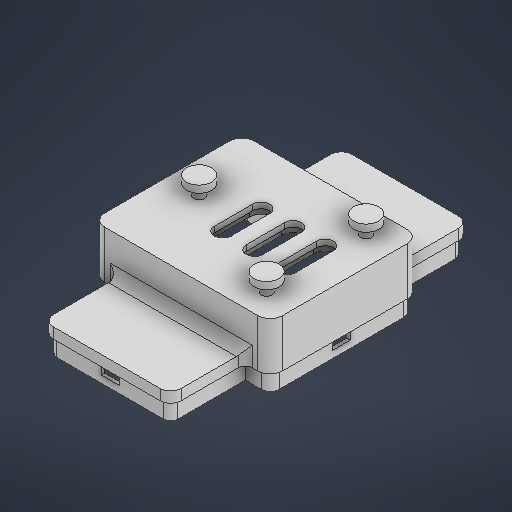
# Autodesk Inventor part: Body_Up
Saved by Autodesk Inventor 2026 (Build 300175000, 175)
## iProperties
Created: 2025-04-18
Part Number: Body_Up
Material: Generic
Document SubType Name: Modeling
Designer: ct_vi
Density: 1 g/cm^3
Appearance: Default
Author: ct_vi
Autodesk Inventor part; units mm, degrees
ref_plane "YZ Plane" through (0, 0, 0) normal (1, 0, 0) x (0, 1, 0)
ref_plane "XZ Plane" through (0, 0, 0) normal (0, 1, 0) x (-1, 0, 0)
ref_plane "XY Plane" through (0, 0, 0) normal (0, 0, 1) x (1, 0, 0)
sketch "Sketch1" plane through (0, 0, 0) normal (0, 1, 0) x (-1, 0, 0)
  line L0 (21.5, 21) -> (-21.5, 21)
  line L1 (-25, 17.5) -> (-25, -17.5)
  line L2 (-21.5, -21) -> (21.5, -21)
  line L3 (25, -17.5) -> (25, 17.5)
  line L4 (25, 21) -> (-25, -21) construction
  line L5 (-25, 21) -> (25, -21) construction
  line L6 (21.5, 20) -> (-21.5, 20)
  line L7 (-24, 17.5) -> (-24, -17.5)
  line L8 (-21.5, -20) -> (21.5, -20)
  line L9 (24, -17.5) -> (24, 17.5)
  line L10 (24, 20) -> (-24, -20) construction
  line L11 (-24, 20) -> (24, -20) construction
  line L12 (-21.5, 19) -> (21.5, 19)
  line L13 (23, 17.5) -> (23, -17.5)
  line L14 (21.5, -19) -> (-21.5, -19)
  line L15 (-23, -17.5) -> (-23, 17.5)
  line L16 (-23, 19) -> (23, -19) construction
  line L17 (23, 19) -> (-23, -19) construction
  line L18 (-22, 18) -> (22, -18) construction
  line L19 (22, 18) -> (-22, -18) construction
  line L20 (36.7273, 0) -> (-33.3361, 0)
  arc A0 (25, 17.5) -> (21.5, 21) centre (21.5, 17.5) ccw
  arc A1 (21.5, -21) -> (25, -17.5) centre (21.5, -17.5) ccw
  arc A2 (-21.5, 21) -> (-25, 17.5) centre (-21.5, 17.5) ccw
  arc A3 (-25, -17.5) -> (-21.5, -21) centre (-21.5, -17.5) ccw
  arc A4 (24, 17.5) -> (21.5, 20) centre (21.5, 17.5) ccw
  arc A5 (21.5, -20) -> (24, -17.5) centre (21.5, -17.5) ccw
  arc A6 (-21.5, 20) -> (-24, 17.5) centre (-21.5, 17.5) ccw
  arc A7 (-24, -17.5) -> (-21.5, -20) centre (-21.5, -17.5) ccw
  arc A8 (23, 17.5) -> (21.5, 19) centre (21.5, 17.5) ccw
  arc A9 (21.5, -19) -> (23, -17.5) centre (21.5, -17.5) ccw
  arc A10 (-23, -17.5) -> (-21.5, -19) centre (-21.5, -17.5) ccw
  arc A11 (-21.5, 19) -> (-23, 17.5) centre (-21.5, 17.5) ccw
  line L21 (-16, 20) -> (-16, 19)
  line L22 (16, 20) -> (16, 19)
  line L23 (-16, -20) -> (-16, -19)
  line L24 (16, -20) -> (16, -19)
  point P0 (0, 0)
  dimension "d0" = 50
  dimension "d1" = 42
  dimension "d2" = 48
  dimension "d3" = 40
  dimension "d4" = 46
  dimension "d5" = 38
  dimension "d27" = 3.5
  dimension "d28" = 2.5
  dimension "d29" = 1.5
  constraints: 50 end point, 29 point on line, 24 point on circle, 24 tangent, 12 centre point, 9 equal radius, 8 midpoint, 7 perpendicular, 6 parallel, 4 horizontal, 2 symmetric about line
  measures "d0" distance of L5.end L4.end
  measures "d1" distance of L4.end L5.start
  measures "d2" distance of L11.end L10.end
  measures "d3" distance of L10.end L11.start
  measures "d4" distance of L16.end L17.end
  measures "d5" distance of L17.start L16.end
  measures "d27" radius of A0
  measures "d28" radius of A4
  measures "d29" radius of A8
extrude "Extrusion1" add sketch "Sketch1" against normal blind 16 contours L20 L13 A8 L12 L22 L6 A4 L9 | L9 A5 L8 L24 L14 A9 L13 L20 | L20 L15 A10 L14 L23 L8 A7 L7 | L7 A6 L6 L21 L12 A11 L15 L20 | L8 L23 L14 L24 | L22 L12 L21 L6
extrude "Extrusion2" add sketch "Sketch1" along normal blind 2.5 and the other way blind 1
extrude "Extrusion5" add sketch "Sketch1" against normal blind 11 contours A0 L3 L20 L9 A4 L6 A6 L7 L1 A2 L0 | L3 A1 L2 A3 L1 L20 L7 A7 L8 A5 L9
sketch "Sketch7" plane through (0, -1, 0) normal (0, -1, 0) x (1, 0, 0)
  line L0 (14, -8.55) -> (14, -8.55)
  line L1 (17.15, -5.4) -> (17.15, 5.4)
  line L2 (14, 8.55) -> (14, 8.55)
  line L3 (10.85, 5.4) -> (10.85, -5.4)
  line L4 (10.85, -8.55) -> (17.15, 8.55) construction
  line L5 (17.15, -8.55) -> (10.85, 8.55) construction
  line L6 (5, -8.5739) -> (5, -8.5739)
  line L7 (8.15, -5.4239) -> (8.15, 5.3761)
  line L8 (5, 8.5261) -> (5, 8.5261)
  line L9 (1.85, 5.3761) -> (1.85, -5.4239)
  line L10 (1.85, -8.5739) -> (8.15, 8.5261) construction
  line L11 (8.15, -8.5739) -> (1.85, 8.5261) construction
  line L12 (5, -0.0239) -> (-4, -0.0239)
  line L13 (-4, -8.5739) -> (-4, -8.5739)
  line L14 (-0.85, -5.4239) -> (-0.85, 5.3761)
  line L15 (-4, 8.5261) -> (-4, 8.5261)
  line L16 (-7.15, 5.3761) -> (-7.15, -5.4239)
  line L17 (-7.15, -8.5739) -> (-0.85, 8.5261) construction
  line L18 (-0.85, -8.5739) -> (-7.15, 8.5261) construction
  arc A0 (-7.15, -5.4239) -> (-4, -8.5739) centre (-4, -5.4239) ccw
  arc A1 (-4, -8.5739) -> (-0.85, -5.4239) centre (-4, -5.4239) ccw
  arc A2 (-4, 8.5261) -> (-7.15, 5.3761) centre (-4, 5.3761) ccw
  arc A3 (-0.85, 5.3761) -> (-4, 8.5261) centre (-4, 5.3761) ccw
  arc A4 (1.85, -5.4239) -> (5, -8.5739) centre (5, -5.4239) ccw
  arc A5 (5, -8.5739) -> (8.15, -5.4239) centre (5, -5.4239) ccw
  arc A6 (8.15, 5.3761) -> (5, 8.5261) centre (5, 5.3761) ccw
  arc A7 (5, 8.5261) -> (1.85, 5.3761) centre (5, 5.3761) ccw
  arc A8 (10.85, -5.4) -> (14, -8.55) centre (14, -5.4) ccw
  arc A9 (14, -8.55) -> (17.15, -5.4) centre (14, -5.4) ccw
  arc A10 (17.15, 5.4) -> (14, 8.55) centre (14, 5.4) ccw
  arc A11 (14, 8.55) -> (10.85, 5.4) centre (14, 5.4) ccw
  line L19 (-4, 7.7261) -> (-4, 7.7261)
  line L20 (-1.65, 5.3761) -> (-1.65, -5.4239)
  line L21 (-4, -7.7739) -> (-4, -7.7739)
  line L22 (-6.35, -5.4239) -> (-6.35, 5.3761)
  line L23 (-6.35, 7.7261) -> (-1.65, -7.7739) construction
  line L24 (-1.65, 7.7261) -> (-6.35, -7.7739) construction
  line L25 (5, -7.7739) -> (5, -7.7739)
  line L26 (7.35, -5.4239) -> (7.35, 5.3761)
  line L27 (5, 7.7261) -> (5, 7.7261)
  line L28 (2.65, 5.3761) -> (2.65, -5.4239)
  line L29 (2.65, -7.7739) -> (7.35, 7.7261) construction
  line L30 (7.35, -7.7739) -> (2.65, 7.7261) construction
  line L31 (14, -7.75) -> (14, -7.75)
  line L32 (16.35, -5.4) -> (16.35, 5.4)
  line L33 (14, 7.75) -> (14, 7.75)
  line L34 (11.65, 5.4) -> (11.65, -5.4)
  line L35 (11.65, -7.75) -> (16.35, 7.75) construction
  line L36 (16.35, -7.75) -> (11.65, 7.75) construction
  arc A12 (-6.35, -5.4239) -> (-4, -7.7739) centre (-4, -5.4239) ccw
  arc A13 (-4, -7.7739) -> (-1.65, -5.4239) centre (-4, -5.4239) ccw
  arc A14 (-1.65, 5.3761) -> (-4, 7.7261) centre (-4, 5.3761) ccw
  arc A15 (-4, 7.7261) -> (-6.35, 5.3761) centre (-4, 5.3761) ccw
  arc A16 (2.65, -5.4239) -> (5, -7.7739) centre (5, -5.4239) ccw
  arc A17 (5, -7.7739) -> (7.35, -5.4239) centre (5, -5.4239) ccw
  arc A18 (7.35, 5.3761) -> (5, 7.7261) centre (5, 5.3761) ccw
  arc A19 (5, 7.7261) -> (2.65, 5.3761) centre (5, 5.3761) ccw
  arc A20 (11.65, -5.4) -> (14, -7.75) centre (14, -5.4) ccw
  arc A21 (14, -7.75) -> (16.35, -5.4) centre (14, -5.4) ccw
  arc A22 (16.35, 5.4) -> (14, 7.75) centre (14, 5.4) ccw
  arc A23 (14, 7.75) -> (11.65, 5.4) centre (14, 5.4) ccw
  point P0 (14, 0)
  point P1 (-4, -0.0239)
  point P2 (5, 8.5261)
  dimension "d99" = 6.3
  dimension "d100" = 17.1
  dimension "d102" = 6.3
  dimension "d103" = 17.1
  dimension "d105" = 9
  dimension "d106" = 6.3
  dimension "d107" = 17.1
  dimension "d108" = 3.15
  dimension "d109" = 4.7
  dimension "d110" = 15.5
  dimension "d111" = 4.7
  dimension "d112" = 15.5
  dimension "d113" = 4.7
  dimension "d114" = 15.5
  dimension "d115" = 2.35
  constraints: 74 end point, 48 point on circle, 48 point on line, 48 tangent, 24 centre point, 22 equal radius, 12 parallel, 10 midpoint, 7 horizontal, 6 perpendicular
  measures "d99" distance of L5.end L4.end
  measures "d100" distance of L4.end L5.start
  measures "d102" distance of L11.end L10.end
  measures "d103" distance of L10.end L11.start
  measures "d105" distance of L12.start L12.end
  measures "d106" distance of L18.end L17.end
  measures "d107" distance of L17.end L18.start
  measures "d108" radius of A0
  measures "d109" distance of L23.end L24.end
  measures "d110" distance of L24.start L23.end
  measures "d111" distance of L30.end L29.end
  measures "d112" distance of L29.end L30.start
  measures "d113" distance of L36.end L35.end
  measures "d114" distance of L35.end L36.start
  measures "d115" radius of A12
ref_plane "Work Plane4" through (0, -8, 0) normal (0, -1, 0) x (1, 0, 0)
sketch "Sketch11" plane through (0, -8, 0) normal (0, -1, 0) x (1, 0, 0)
  line L0 (0, 42) -> (-15, 42)
  line L1 (0, 42) -> (0, 41)
  line L2 (0, 41) -> (-15, 41)
  line L3 (0, 41) -> (0, 40)
  line L4 (0, 40) -> (-15, 40)
  line L5 (-18, 39) -> (-18, 20)
  line L6 (-17, 39) -> (-17, 20)
  line L7 (-16, 39) -> (-16, 19)
  line L8 (0, 21) -> (0, 42)
  line L9 (-18, 20) -> (0, 20)
  arc A0 (-15, 40) -> (-16, 39) centre (-15, 39) ccw
  arc A1 (-15, 41) -> (-17, 39) centre (-15, 39) ccw
  arc A2 (-15, 42) -> (-18, 39) centre (-15, 39) ccw
  line L10 (0, 0) -> (0, 21)
  line L11 (-16, 19) -> (0, 19)
  line L12 (-17, 20) -> (-17, 19)
  line L13 (-17, 19) -> (-16, 19)
  line L14 (-0.3234, 0) -> (-24.4289, 0)
  line L15 (-17, -19) -> (-16, -19)
  line L16 (-16, -19) -> (0, -19)
  line L17 (-17, -20) -> (-17, -19)
  line L18 (-18, -20) -> (0, -20)
  line L19 (-16, -39) -> (-16, -19)
  line L20 (-17, -39) -> (-17, -20)
  line L21 (-18, -39) -> (-18, -20)
  arc A3 (-17, -39) -> (-15, -41) centre (-15, -39) ccw
  arc A4 (-18, -39) -> (-15, -42) centre (-15, -39) ccw
  line L22 (0, -40) -> (-15, -40)
  line L23 (0, -41) -> (-15, -41)
  line L24 (0, -42) -> (0, -41)
  line L25 (0, -42) -> (-15, -42)
  arc A5 (-16, -39) -> (-15, -40) centre (-15, -39) ccw
  line L26 (17, -19) -> (16, -19)
  line L27 (17, -20) -> (17, -19)
  line L28 (16, -19) -> (0, -19)
  line L29 (18, -20) -> (0, -20)
  line L30 (16, -39) -> (16, -19)
  line L31 (18, -39) -> (18, -20)
  line L32 (17, -39) -> (17, -20)
  line L33 (0, 40) -> (15, 40)
  line L34 (0, 41) -> (15, 41)
  line L35 (0, 42) -> (15, 42)
  arc A6 (16, 39) -> (15, 40) centre (15, 39) ccw
  arc A7 (17, 39) -> (15, 41) centre (15, 39) ccw
  arc A8 (18, 39) -> (15, 42) centre (15, 39) ccw
  line L36 (16, 39) -> (16, 19)
  line L37 (17, 39) -> (17, 20)
  line L38 (18, 39) -> (18, 20)
  line L39 (16, 19) -> (0, 19)
  line L40 (18, 20) -> (0, 20)
  line L41 (17, 19) -> (16, 19)
  line L42 (17, 20) -> (17, 19)
  line L43 (0, -40) -> (15, -40)
  line L44 (0, -41) -> (15, -41)
  line L45 (0, -42) -> (15, -42)
  arc A9 (15, -40) -> (16, -39) centre (15, -39) ccw
  arc A10 (15, -41) -> (17, -39) centre (15, -39) ccw
  arc A11 (15, -42) -> (18, -39) centre (15, -39) ccw
  line L46 (0, -41) -> (0, -40)
  point P0 (0, 0)
  point P1 (0, 0)
  point P2 (-18, 42)
  point P3 (-17, 41)
  point P4 (-16, 40)
  point P5 (-16, -40)
  point P6 (-17, -41)
  point P7 (-18, -42)
  point P8 (0, -21)
  point P9 (16, -40)
  point P10 (18, -42)
  point P11 (17, -41)
  point P12 (16, 40)
  point P13 (17, 41)
  point P14 (18, 42)
  point P15 (16, 20)
  point P16 (-16, 20)
  point P17 (16, -20)
  point P18 (-16, -20)
  dimension "d127" = 21
  dimension "d128" = 21
  dimension "d129" = 18
  dimension "d130" = 90
  dimension "d131" = 22
  dimension "d132" = 1
  dimension "d133" = 17
  dimension "d134" = 90
  dimension "d135" = 1
  dimension "d136" = 16
  dimension "d137" = 21
  dimension "d138" = 3
  dimension "d139" = 2
  dimension "d140" = 1
  constraints: 94 end point, 54 symmetric about line, 32 point on line, 24 point on circle, 12 centre point, 9 perpendicular, 6 tangent, 2 vertical, 1 horizontal, 9 other
  measures "d127" distance of L10.start L8.start
  measures "d128" distance of L8.start L0.start
  measures "d129" distance of L0.start point (-18, 42)
  measures "d130" angle of L0 L8
  measures "d131" distance of point (-18, 42) L9.start
  measures "d132" distance of L0.start L2.start
  measures "d133" distance of L2.start point (-17, 41)
  measures "d134" angle of L1 L2
  measures "d135" distance of L2.start L4.start
  measures "d136" distance of L4.start point (-16, 40)
  measures "d137" distance of point (-16, 40) L13.end
  measures "d138" radius of A2
  measures "d139" radius of A1
  measures "d140" radius of A0
extrude "Extrusion14" cut sketch "Sketch7" against normal blind 1.9
extrude "Extrusion15" cut sketch "Sketch7" against normal through all contours L20 A13 A12 L22 A15 A14 | A17 A16 L28 A19 A18 L26 | A21 A20 L34 A23 A22 L32
extrude "Extrusion16" add sketch "Sketch11" along normal blind 1.5 contours L1 L2 A1 L6 L9 L5 A2 L0 | L35 A8 L38 L40 L37 A7 L34 L1 | L3 L4 A0 L7 L9 L6 A1 L2 | L34 A7 L37 L40 L36 A6 L33 L3 | L8 L10 L9 L7 A0 L4 | L33 A6 L36 L40 L10 L8 | L20 A3 L23 L24 L25 A4 L21 L18 | L18 L19 A5 L22 L46 L23 A3 L20 | L18 L29 L30 A9 L43 L22 A5 L19 | L29 L32 A10 L44 L46 L43 A9 L30 | L44 A10 L32 L29 L31 A11 L45 L24
extrude "Extrusion17" add sketch "Sketch11" along normal blind 3 contours L1 L2 A1 L6 L9 L5 A2 L0 | L35 A8 L38 L40 L37 A7 L34 L1 | L20 A3 L23 L24 L25 A4 L21 L18 | L44 A10 L32 L29 L31 A11 L45 L24
extrude "Extrusion18" add sketch "Sketch11" along normal blind 8 contours L3 L4 A0 L7 L9 L6 A1 L2 | L34 A7 L37 L40 L36 A6 L33 L3 | L18 L19 A5 L22 L46 L23 A3 L20 | L29 L32 A10 L44 L46 L43 A9 L30
sketch "Sketch12" plane through (16, -16, -20) normal (0, 0, -1) x (-1, 0, 0)
  line L0 (0, 5) -> (0, 0) projected
  line L1 (37.5, 0) -> (-5.5, 0) projected
  line L2 (0, 5) -> (32, 5)
  line L3 (32, 5) -> (32, 0)
  line L4 (32, 0) -> (0, 0)
  line L5 (0, 0) -> (0, 5)
  point P0 (16, 16)
  constraints: 8 end point, 2 parallel, 1 horizontal, 1 perpendicular
extrude "Extrusion19" cut sketch "Sketch12" against normal up to surface (40 mm away)
sketch "Sketch13" plane through (0, -9.5, 0) normal (0, -1, 0) x (1, 0, 0)
  line L0 (21.7839, 0) -> (0, 0)
  line L1 (0, 0) -> (0, 35.5)
  line L2 (-14, 37) -> (14, 37)
  line L3 (14, 37) -> (14, 34)
  line L4 (14, 34) -> (-14, 34)
  line L5 (-14, 34) -> (-14, 37)
  line L6 (-14, 37) -> (14, 34) construction
  line L7 (14, 37) -> (-14, 34) construction
  line L8 (-14, -37) -> (14, -37)
  line L9 (14, -37) -> (14, -34)
  line L10 (14, -34) -> (-14, -34)
  line L11 (-14, -34) -> (-14, -37)
  line L12 (-14, -37) -> (14, -34) construction
  line L13 (14, -37) -> (-14, -34) construction
  point P0 (0, -35.5)
  dimension "d153" = 28
  dimension "d154" = 3
  dimension "d155" = 35.5
  constraints: 28 end point, 5 symmetric about line, 2 horizontal, 2 midpoint, 2 parallel, 2 perpendicular
  measures "d153" distance of L3.end L4.end
  measures "d154" distance of L2.end L3.end
  measures "d155" distance of L0.end L1.end
extrude "Extrusion20" add sketch "Sketch13" along normal blind 3.9
fillet "Fillet1" radius 1.5 8 edges at (-14, -11.45, 37) (-14, -11.45, 34) (14, -11.45, 34) (14, -11.45, 37) (-14, -11.45, -34) (-14, -11.45, -37) (14, -11.45, -34) (14, -11.45, -37)
fillet "Fillet2" radius 1.5 12 edges at (15.7071, -9.5, -39.7071) (0, -9.5, -40) (-15.7071, -9.5, -39.7071) (-16, -9.5, -30) (16, -9.5, -30) (0, -9.5, -21) (15.7071, -9.5, 39.7071) (0, -9.5, 40) (-15.7071, -9.5, 39.7071) (-16, -9.5, 30) (16, -9.5, 30) (0, -9.5, 21)
fillet "Fillet3" radius 2 8 edges at (22.5607, -1, 18.5607) (23, -1, 0) (22.5607, -1, -18.5607) (0, -1, -19) (-22.5607, -1, -18.5607) (-23, -1, 0) (-22.5607, -1, 18.5607) (0, -1, 19)
fillet "Fillet4" radius 2 4 edges at (18, -9.5, 21) (18, -9.5, -21) (-18, -9.5, -21) (-18, -9.5, 21)
fillet "Fillet5" radius 2.5 6 edges at (-19, -8, -21) (0, -8, -21) (19, -8, -21) (-19, -8, 21) (0, -8, 21) (19, -8, 21)
sketch "Sketch14" plane through (15, -11, -41) normal (0, 0, -1) x (-1, 0, 0)
  line L0 (0, 0) -> (0, -5) projected
  line L1 (0, 0) -> (15, 0)
  line L2 (30, 0) -> (0, 0) projected
  line L3 (15, 0) -> (15, -2)
  line L4 (12.5, -1) -> (17.5, -1)
  line L5 (17.5, -1) -> (17.5, -3)
  line L6 (17.5, -3) -> (12.5, -3)
  line L7 (12.5, -3) -> (12.5, -1)
  line L8 (12.5, -1) -> (17.5, -3) construction
  line L9 (17.5, -1) -> (12.5, -3) construction
  point P0 (15, 11)
  dimension "d163" = 15
  dimension "d164" = 2
  dimension "d165" = 5
  dimension "d166" = 2
  constraints: 16 end point, 3 midpoint, 2 parallel, 2 perpendicular, 1 horizontal
  measures "d163" distance of L0.start L1.end
  measures "d164" distance of L1.end L3.end
  measures "d165" distance of L5.end L6.end
  measures "d166" distance of L4.end L5.end
extrude "Extrusion21" cut sketch "Sketch14" against normal up to surface (1 mm away)
sketch "Sketch15" plane through (-15, -11, 41) normal (0, 0, 1) x (1, 0, 0)
  line L0 (0, 0) -> (-2, 0) projected
  line L1 (0, 0) -> (15, 0)
  line L2 (0, 0) -> (30, 0) projected
  line L3 (0, 0) -> (15, 0) construction
  line L4 (15, 0) -> (15, -2)
  line L5 (12.5, -1) -> (17.5, -1)
  line L6 (17.5, -1) -> (17.5, -3)
  line L7 (17.5, -3) -> (12.5, -3)
  line L8 (12.5, -3) -> (12.5, -1)
  line L9 (12.5, -1) -> (17.5, -3) construction
  line L10 (17.5, -1) -> (12.5, -3) construction
  point P0 (15, 11)
  dimension "d127" = 21
  dimension "d130" = 90
  dimension "d134" = 90
  dimension "d169" = 15
  dimension "d170" = 0
  dimension "d171" = 2
  dimension "d172" = 5
  dimension "d173" = 2
  constraints: 18 end point, 2 collinear, 2 horizontal, 2 midpoint, 2 parallel, 2 perpendicular
  measures "d169" distance of L0.start L1.end
  measures "d170" distance between parallel lines of L1 L3
  measures "d171" distance of L1.end L4.end
  measures "d172" distance of L6.end L7.end
  measures "d173" distance of L5.end L6.end
extrude "Extrusion22" cut sketch "Sketch15" against normal up to surface (1 mm away)
sketch "Sketch16" plane through (-24, -16, -17.5) normal (-1, 0, 0) x (0, 0, 1)
  line L0 (35, 5) -> (0, 5) projected
  line L1 (0, 5) -> (17.5, 5)
  line L2 (0, 5) -> (17.5, 5) construction
  line L3 (17.5, 5) -> (17.5, 3)
  line L4 (20, 2) -> (15, 2)
  line L5 (15, 2) -> (15, 4)
  line L6 (15, 4) -> (20, 4)
  line L7 (20, 4) -> (20, 2)
  line L8 (20, 2) -> (15, 4) construction
  line L9 (15, 2) -> (20, 4) construction
  point P0 (17.5, 16)
  dimension "d176" = 17.5
  dimension "d177" = 0
  dimension "d178" = 2
  dimension "d179" = 5
  dimension "d180" = 2
  constraints: 18 end point, 2 collinear, 2 horizontal, 2 midpoint, 2 parallel, 2 perpendicular
  measures "d176" distance of L0.end L1.end
  measures "d177" distance between parallel lines of L1 L2
  measures "d178" distance of L1.end L3.end
  measures "d179" distance of L5.end L6.end
  measures "d180" distance of L4.end L5.end
extrude "Extrusion23" cut sketch "Sketch16" against normal through all
sketch "Sketch17" plane through (0, -1, 0) normal (0, -1, 0) x (1, 0, 0)
  line L0 (0, 0) -> (-16, 0)
  line L1 (-16, 0) -> (-16, -11)
  circle A0 centre (-16, -11) radius 3
  line L2 (-16, 0) -> (-16, 11)
  circle A1 centre (-16, 11) radius 3
  circle A2 centre (-16, -11) radius 3.5
  circle A3 centre (-16, 11) radius 3.5
  dimension "d183" = 16
  dimension "d184" = 11
  dimension "d185" = 6
  dimension "d186" = 11
  dimension "d187" = 6
  dimension "d188" = 7
  dimension "d189" = 7
  constraints: 6 end point, 4 centre point, 4 coincident, 1 horizontal, 1 perpendicular, 1 vertical
  measures "d183" distance of L0.start L0.end
  measures "d184" distance of L0.end L1.end
  measures "d185" diameter of A0
  measures "d186" distance of L0.end L2.end
  measures "d187" diameter of A1
  measures "d188" diameter of A2
  measures "d189" diameter of A3
extrude "Extrusion24" add sketch "Sketch17" along normal blind 2
extrude "Extrusion25" cut sketch "Sketch17" against normal blind 1.5 contours A0 | A1
ref_plane "Work Plane5" through (-16, -11, -15) normal (0, 0, 1) x (1, 0, 0)
sketch "Sketch19" plane through (-16, -11, -15) normal (0, 0, 1) x (1, 0, 0)
  line L0 (0, 0) -> (0, 8)
  line L1 (-3.5, 8) -> (3.5, 8) projected
  line L2 (0, 8) -> (-1, 8)
  line L3 (-1, 8) -> (1, 8)
  line L4 (1, 8) -> (1, 9.5)
  line L5 (1, 9.5) -> (-1, 9.5)
  line L6 (-1, 9.5) -> (-1, 8)
  point P0 (16, 11)
  dimension "d195" = 1
  dimension "d196" = 2
  dimension "d197" = 1.5
  constraints: 12 end point, 2 parallel, 2 perpendicular, 1 horizontal, 1 midpoint
  measures "d195" distance of L0.end L2.end
  measures "d196" distance of L5.end L4.end
  measures "d197" distance of L4.end L3.end
extrude "Extrusion26" cut sketch "Sketch19" along normal blind 31.25
sketch "Sketch20" plane through (0, 2.5, 0) normal (0, 1, 0) x (1, 0, 0)
  line L0 (0, 0) -> (-16, 0)
  line L1 (0, 0) -> (17, 0)
  line L2 (17, 0) -> (17, -14)
  circle A0 centre (17, -14) radius 3.5
  circle A1 centre (17, -14) radius 1.5
  circle A2 centre (17, 14) radius 3.5
  circle A3 centre (17, 14) radius 1.5
  circle A4 centre (-16, 0) radius 3.5
  circle A5 centre (-16, 0) radius 1.5
  dimension "d200" = 16
  dimension "d201" = 17
  dimension "d202" = 14
  dimension "d203" = 7
  dimension "d204" = 3
  dimension "d205" = 7
  dimension "d206" = 3
  constraints: 6 centre point, 6 coincident, 6 end point, 3 symmetric about line, 2 horizontal, 1 perpendicular, 2 other
  measures "d200" distance of L0.start L0.end
  measures "d201" distance of L0.start L1.end
  measures "d202" distance of L1.end L2.end
  measures "d203" diameter of A0
  measures "d204" diameter of A1
  measures "d205" diameter of A4
  measures "d206" diameter of A5
extrude "Extrusion27" add sketch "Sketch20" along normal blind 3 contours A1 | A3 | A5
ref_plane "Work Plane6" through (0, 5.5, 0) normal (0, 1, 0) x (1, 0, 0)
sketch "Sketch21" plane through (0, 5.5, 0) normal (0, 1, 0) x (1, 0, 0)
  line L0 (0, 0) -> (17, 0)
  circle A0 centre (17, -14) radius 1.5 projected
  line L1 (17, 0) -> (17, -14)
  circle A1 centre (17, -14) radius 3.5
  circle A2 centre (17, 14) radius 1.5
  circle A3 centre (17, 14) radius 3.5
  line L2 (0, 0) -> (-16, 0)
  line L3 (0, 0) -> (16, 0) construction
  circle A4 centre (-16, 0) radius 3.5
  dimension "d210" = 17
  dimension "d211" = 7
  dimension "d212" = 16
  dimension "d213" = 180
  dimension "d214" = 7
  constraints: 8 end point, 4 centre point, 3 coincident, 3 horizontal, 2 symmetric about line, 1 collinear, 2 other
  measures "d210" distance of L0.start L0.end
  measures "d211" diameter of A1
  measures "d212" distance of L0.start L2.end
  measures "d213" angle of L2 L3
  measures "d214" diameter of A4
extrude "Extrusion28" add sketch "Sketch21" along normal blind 2 contours A0 | A1 | A2 | A3 | A4
body "Solid1"
